Wohnmobil Regal Norbert (Autodesk Fusion 360 design; units mm, degrees)
Autodesk Fusion 360 part; units mm, degrees
sketch "Sketch1" plane through (0, 0, 0) normal (1, 0, 0) x (0, 1, 0)
  line L0 (0, 0) -> (91.3, 0)
  line L1 (91.3, 0) -> (91.3, 81.3)
  line L2 (91.3, 81.3) -> (0, 81.3)
  line L3 (0, 81.3) -> (0, 0)
  line L4 (8, 73.3) -> (83.3, 73.3)
  line L5 (83.3, 73.3) -> (83.3, 8)
  line L6 (83.3, 8) -> (8, 8)
  line L7 (8, 8) -> (8, 73.3)
  circle A0 centre (4, 77.3) radius 1.65
  circle A1 centre (87.3, 77.3) radius 1.65
  circle A2 centre (9.65, 4) radius 1.65
  circle A3 centre (81.65, 4) radius 1.65
  line L8 (0, 44.65) -> (91.3, 44.65)
  line L9 (91.3, 44.65) -> (91.3, 36.65)
  line L10 (91.3, 36.65) -> (0, 36.65)
  line L11 (0, 36.65) -> (0, 44.65)
  circle A4 centre (87.3, 40.65) radius 1.65
  circle A5 centre (33.65, 4) radius 1.65
  line L12 (45.65, 8) -> (45.65, 0)
  circle A6 centre (57.65, 4) radius 1.65
  point P0 (0, 40.65)
  point P1 (0, 40.65)
  point P2 (45.65, 0)
  point P3 (45.65, 81.3)
  point P4 (45.65, 8)
  point P5 (45.65, 4)
  dimension "d6" = 8
  dimension "d7" = 8
  dimension "d8" = 8
  dimension "d9" = 8
  dimension "d10" = 3.3
  dimension "d11" = 91.3
  dimension "d12" = 3.3
  dimension "d13" = 4
  dimension "d14" = 4
  dimension "d15" = 4
  dimension "d16" = 4
  dimension "d17" = 81.3
  dimension "d18" = 3.3
  dimension "d19" = 3.3
  dimension "d20" = 9.65
  dimension "d21" = 4
  dimension "d22" = 9.65
  dimension "d23" = 4
  dimension "d24" = 8
  dimension "d25" = 3.3
  dimension "d26" = 4
  dimension "d27" = 4
  dimension "d64" = 3.3
  dimension "d76" = 3.3
  dimension "d77" = 4
  dimension "d78" = 4
  dimension "d79" = 24
  dimension "d80" = 24
  constraint horizontal L0
  constraint vertical L1
  constraint horizontal L2
  constraint vertical L3
  constraint coincident L0.start L3.end
  constraint horizontal L4
  constraint vertical L5
  constraint horizontal L6
  constraint vertical L7
  constraint horizontal L8
  constraint vertical L9
  constraint horizontal L10
  constraint vertical L11
  constraint coincident L3 L8.start
  constraint coincident L1 L8.end
  constraint midpoint L11 P1
  constraint midpoint L3 P1
  constraint coincident P1 P0
  constraint midpoint L0 P2
  constraint midpoint L2 P3
  constraint midpoint L6 P4
  constraint coincident P4 L12.start
  constraint coincident P2 L12.end
  constraint midpoint L12 P5
  measures "d6" distance of L2 L4
  measures "d7" distance of L1 L5
  measures "d8" distance of L0 L6
  measures "d9" distance of L3 L7
  measures "d10" diameter of A0
  measures "d11" distance of L1.end L2.end
  measures "d12" diameter of A1
  measures "d13" distance of L2 A0.centre
  measures "d14" distance of L3 A0.centre
  measures "d15" distance of L1 A1.centre
  measures "d16" distance of L2 A1.centre
  measures "d17" distance of L0.end L1.end
  measures "d18" diameter of A2
  measures "d19" diameter of A3
  measures "d20" distance of L1 A3.centre
  measures "d21" distance of L0 A3.centre
  measures "d22" distance of L3 A2.centre
  measures "d23" distance of L0 A2.centre
  measures "d24" distance of L8.start L10.end
  measures "d25" diameter of A4
  measures "d26" distance of L1 A4.centre
  measures "d27" distance of L8 A4.centre
  measures "d64" diameter of A5
  measures "d76" diameter of A6
  measures "d77" distance of L0 A5.centre
  measures "d78" distance of L0 A6.centre
  measures "d79" distance of A2.centre A5.centre
  measures "d80" distance of A3.centre A6.centre
extrude "Extrude1" add sketch "Sketch1" along normal blind 8 contours L0 L3 L6 L7 L10 L12 | L0 L1 L5 L6 L10 L12 | L3 L7 L8 L10 L11 | L1 L2 L3 L4 L5 L7 L8 | L5 L7 L8 L10 | L1 L5 L8 L9 L10 | A0 | A1 | A2 | A3 | A4 | A5 | A6 makes body 1
extrude "Extrude2" cut sketch "Sketch1" along normal blind 8 from surface at 3 contours A0 | A1 | A2 | A3 | A4 | A5 | A6 bodies 1
sketch "Sketch2" plane through (0, 0, 0) normal (-1, 0, 0) x (0, -1, 0)
  line L0 (-83.3, 36.65) -> (-8, 36.65)
  line L1 (-8, 36.65) -> (-8, 8)
  line L2 (-8, 8) -> (-83.3, 8)
  line L3 (-83.3, 8) -> (-83.3, 36.65)
  line L4 (-8, 44.65) -> (-83.3, 44.65)
  line L5 (-83.3, 44.65) -> (-83.3, 73.3)
  line L6 (-83.3, 73.3) -> (-8, 73.3)
  line L7 (-8, 73.3) -> (-8, 44.65)
  line L8 (-91.3, 0) -> (0, 0)
  line L9 (0, 0) -> (0, 81.3)
  line L10 (0, 81.3) -> (-91.3, 81.3)
  line L11 (-91.3, 81.3) -> (-91.3, 0)
  line L12 (0, 81.3) -> (-4, 81.3)
  line L13 (-4, 81.3) -> (-4, 71.3)
  line L14 (-4, 71.3) -> (0, 71.3)
  line L15 (0, 71.3) -> (0, 81.3)
  line L16 (0, 0) -> (-4, 0)
  line L17 (-4, 0) -> (-4, 10)
  line L18 (-4, 10) -> (0, 10)
  line L19 (0, 10) -> (0, 0)
  dimension "d33" = 4
  dimension "d34" = 10
  dimension "d35" = 4
  dimension "d36" = 10
  constraint horizontal L12
  constraint vertical L13
  constraint horizontal L14
  constraint vertical L15
  constraint coincident L9.end L10.start
  constraint horizontal L16
  constraint vertical L17
  constraint horizontal L18
  constraint vertical L19
  constraint coincident L8.end L9.start
  measures "d33" distance of L9.end L12.end
  measures "d34" distance of L9.end L14.end
  measures "d35" distance of L8.end L16.end
  measures "d36" distance of L8.end L18.end
extrude "Extrude3" add sketch "Sketch2" along normal blind 10 contours L8 L9 L16 L17 L18 L19 | L9 L10 L12 L13 L14 L15 bodies 1
sketch "Sketch3" plane through (0, 4, 0) normal (0, 1, 0) x (-1, 0, 0)
  line L0 (0, 81.3) -> (0, 71.3)
  line L1 (0, 71.3) -> (10, 71.3)
  line L2 (10, 71.3) -> (10, 81.3)
  line L3 (10, 81.3) -> (0, 81.3)
  circle A0 centre (5, 76.3) radius 2
  circle A1 centre (5, 5) radius 2
  line L4 (0, 10) -> (10, 10)
  line L5 (10, 10) -> (10, 0)
  dimension "d39" = 4
  dimension "d40" = 5
  dimension "d41" = 5
  dimension "d42" = 4
  dimension "d43" = 5
  dimension "d44" = 5
  measures "d39" diameter of A0
  measures "d40" distance of L3 A0.centre
  measures "d41" distance of L2 A0.centre
  measures "d42" diameter of A1
  measures "d43" distance of A1.centre L4
  measures "d44" distance of A1.centre L5
extrude "Extrude4" cut sketch "Sketch3" against normal blind 50 contours A0 | A1 bodies 1
fillet "Fillet1" radius 4 2 edges at (4, 91.3, 81.3) (4, 91.3, 0) on bodies 1
fillet "Fillet2" radius 2 18 edges at (0, 45.65, 44.65) (8, 45.65, 44.65) (0, 45.65, 8) (8, 45.65, 8) (0, 45.65, 73.3) (0, 45.65, 0) (0, 90.1284, 1.1716) (0, 91.3, 40.65) (0, 90.1284, 80.1284) (0, 45.65, 81.3) (8, 43.65, 0) (8, 90.1284, 1.1716) (8, 91.3, 40.65) (8, 90.1284, 80.1284) (8, 43.65, 81.3) (8, 45.65, 73.3) (0, 45.65, 36.65) (8, 45.65, 36.65) on bodies 1
fillet "Fillet3" radius 4 4 edges at (-10, 2, 81.3) (-10, 2, 71.3) (-10, 2, 0) (-10, 2, 10) on bodies 1
sketch "Sketch4" plane through (0, 0, 0) normal (0, 1, 0) x (1, 0, 0)
  line L0 (150.5, 0.7217) -> (122.5193, 0.7217)
  line L1 (122.5193, 0.7217) -> (122.5193, -11.4742)
  line L2 (122.5193, -11.4742) -> (150.5, -11.4742)
  line L3 (150.5, -11.4742) -> (150.5, 0.7217)
  circle A0 centre (146.2185, -7.4747) radius 1.65
  circle A1 centre (140.1985, -5.9111) radius 1.6
  circle A2 centre (133.7541, -4.8359) radius 1.55
  circle A3 centre (127.3283, -3.6191) radius 1.5
  dimension "d55" = 3.3
  dimension "d56" = 3.2
  dimension "d57" = 3.1
  dimension "d58" = 3
  constraint horizontal L0
  constraint vertical L1
  constraint horizontal L2
  constraint vertical L3
  measures "d55" diameter of A0
  measures "d56" diameter of A1
  measures "d57" diameter of A2
  measures "d58" diameter of A3
extrude "Extrude5" add sketch "Sketch4" along normal blind 6 separate body contours L0 L1 L2 L3 | A0 | A1 | A2 | A3 makes body 2
extrude "Extrude6" cut sketch "Sketch4" along normal blind 3 from surface at 3 contours A0 | A1 | A2 | A3 bodies 2
fillet "Fillet4" radius 2 4 edges at (0, 4, 75.3) (0.5858, 4, 80.7142) (0.5858, 4, 0.5858) (0, 4, 6) on bodies 1
fillet "Fillet5" radius 2 2 edges at (0, 3, 71.3) (0, 3, 10) on bodies 1
hidden bodies 2
equation "breite = 80 mm"
equation "hoehe = 70 mm"
equation "bohrung = 3.3 mm"
equation "wandloch = 4 mm"
equation "dicke = 8 mm"
equation "d6 = dicke"
equation "d7 = dicke"
equation "d8 = dicke"
equation "d9 = dicke"
equation "d10 = bohrung"
equation "d11 = breite + ( 2 * bohrung ) + ( dicke - bohrung )"
equation "d12 = bohrung"
equation "d13 = dicke / 2"
equation "d14 = dicke / 2"
equation "d15 = dicke / 2"
equation "d16 = dicke / 2"
equation "d17 = hoehe + ( 2 * bohrung ) + ( dicke - bohrung )"
equation "d18 = bohrung"
equation "d19 = bohrung"
equation "d20 = dicke / 2 + 5.65 mm"
equation "d21 = dicke / 2"
equation "d22 = dicke / 2 + 5.65 mm"
equation "d23 = dicke / 2"
equation "d24 = dicke"
equation "d25 = bohrung"
equation "d26 = dicke / 2"
equation "d27 = dicke / 2"
equation "d28 = dicke"
equation "d30 = dicke / 2 - 1 mm"
equation "d31 = dicke"
equation "d33 = dicke / 2"
equation "d34 = dicke + 2 mm"
equation "d35 = dicke / 2"
equation "d36 = dicke + 2 mm"
equation "d37 = dicke + 2 mm"
equation "d39 = wandloch"
equation "d40 = dicke / 2 + 1 mm"
equation "d41 = dicke / 2 + 1 mm"
equation "d42 = wandloch"
equation "d43 = dicke / 2 + 1 mm"
equation "d44 = dicke / 2 + 1 mm"
equation "d48 = dicke / 2"
equation "d50 = dicke / 4"
equation "d52 = dicke / 2"
equation "d64 = bohrung"
equation "d67 = dicke / 4"
equation "d69 = dicke / 4"
equation "d76 = bohrung"
equation "d77 = dicke / 2"
equation "d78 = dicke / 2"
